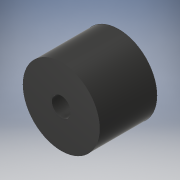
# Autodesk Inventor part: CLB_028_ScissorLiftSpacer
Saved by Autodesk Inventor 2018.3 (Build 223284000, 284)
## iProperties
Created: 2020-01-15
Part Number: CLB_028_ScissorLiftSpacer
Material: Acetal Resin, Black
Document SubType Name: Modeling
Designer: Cooper
Density: 1.425 g/cm^3
Appearance: Smooth - Black
Mass: 1.15347 g
Surface Area: 9.57924 cm^2
Volume: 1.15347 cm^3
Author: Cooper
Autodesk Inventor part; units mm, degrees
ref_plane "YZ Plane" through (0, 0, 0) normal (1, 0, 0) x (0, 1, 0)
ref_plane "XZ Plane" through (0, 0, 0) normal (0, 1, 0) x (-1, 0, 0)
ref_plane "XY Plane" through (0, 0, 0) normal (0, 0, 1) x (1, 0, 0)
sketch "Sketch1" plane through (0, 0, 0) normal (0, 0, 1) x (1, 0, 0)
  circle A0 centre (0, 0) radius 12.7
  circle A1 centre (0, 0) radius 3.175
  dimension "d0" = 25.4
  dimension "d1" = 6.35
  constraints: 2 centre point, 1 coincident
  measures "d0" diameter of A0
  measures "d1" diameter of A1
extrude "Extrusion1" add sketch "Sketch1" along normal blind 19.05
body "Solid1"
